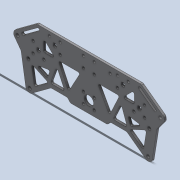
# Autodesk Inventor part: HeadTongueMount2
Saved by Autodesk Inventor 2020 (Build 240168000, 168)
## iProperties
Created: 2021-07-07
Part Number: HeadTongueMount2
Material: Generic
Document SubType Name: Sheet Metal
Designer: Val
Density: 1 g/cm^3
Sheet Metal Rule: Default
Appearance: Default
Author: Val
Autodesk Inventor part; units mm, degrees
ref_plane "YZ Plane" through (0, 0, 0) normal (1, 0, 0) x (0, 1, 0)
ref_plane "XZ Plane" through (0, 0, 0) normal (0, 1, 0) x (-1, 0, 0)
ref_plane "XY Plane" through (0, 0, 0) normal (0, 0, 1) x (1, 0, 0)
sketch "Base" plane through (0, 0, 0) normal (0, 0, 1) x (1, 0, 0)
  line L0 (97.0477, -15.5492) -> (74.2641, 1.2707)
  arc A0 (76.6398, 4.4888) -> (74.2641, 1.2707) centre (75.4519, 2.8798) ccw
  line L1 (76.6398, 4.4888) -> (99.4234, -12.3312)
  arc A1 (97.0477, -15.5492) -> (99.4234, -12.3312) centre (98.2355, -13.9402) ccw
  line L2 (-74.2641, 1.2707) -> (-97.0477, -15.5492)
  arc A2 (-99.4234, -12.3312) -> (-97.0477, -15.5492) centre (-98.2355, -13.9402) ccw
  line L3 (-99.4234, -12.3312) -> (-76.6398, 4.4888)
  arc A3 (-74.2641, 1.2707) -> (-76.6398, 4.4888) centre (-75.4519, 2.8798) ccw
  line L4 (67.5519, -9.1185) -> (67.5519, -20.0701)
  arc A4 (65.5519, -22.0701) -> (67.5519, -20.0701) centre (65.5519, -20.0701) ccw
  line L5 (65.5519, -22.0701) -> (54.6004, -22.0701)
  arc A5 (53.1861, -18.6559) -> (54.6004, -22.0701) centre (54.6004, -20.0701) ccw
  line L6 (53.1861, -18.6559) -> (64.1377, -7.7043)
  arc A6 (67.5519, -9.1185) -> (64.1377, -7.7043) centre (65.5519, -9.1185) ccw
  line L7 (-67.5519, -20.0701) -> (-67.5519, -9.1185)
  arc A7 (-64.1377, -7.7043) -> (-67.5519, -9.1185) centre (-65.5519, -9.1185) ccw
  line L8 (-64.1377, -7.7043) -> (-53.1861, -18.6559)
  arc A8 (-54.6004, -22.0701) -> (-53.1861, -18.6559) centre (-54.6004, -20.0701) ccw
  line L9 (-54.6004, -22.0701) -> (-65.5519, -22.0701)
  arc A9 (-67.5519, -20.0701) -> (-65.5519, -22.0701) centre (-65.5519, -20.0701) ccw
  arc A10 (51.746, -36.138) -> (48.4208, -33.6832) centre (50.0834, -34.9106) ccw
  line L10 (51.746, -36.138) -> (39.6773, -52.4858)
  arc A11 (36.3521, -50.0309) -> (39.6773, -52.4858) centre (38.0147, -51.2583) ccw
  line L11 (36.3521, -50.0309) -> (48.4208, -33.6832)
  arc A12 (26.5915, -49.1395) -> (29.9167, -51.5944) centre (28.2541, -50.3669) ccw
  line L12 (26.5915, -49.1395) -> (41.6774, -28.7049)
  arc A13 (45.0026, -31.1597) -> (41.6774, -28.7049) centre (43.34, -29.9323) ccw
  line L13 (45.0026, -31.1597) -> (29.9167, -51.5944)
  line L14 (74.2192, -47.1822) -> (63.9766, -52.1292)
  arc A14 (61.2238, -51.0023) -> (63.9766, -52.1292) centre (63.1067, -50.3283) ccw
  line L15 (61.2238, -51.0023) -> (58.7121, -43.9862)
  arc A15 (60.9154, -41.338) -> (58.7121, -43.9862) centre (60.5951, -43.3122) ccw
  line L16 (60.9154, -41.338) -> (73.6697, -43.4071)
  arc A16 (74.2192, -47.1822) -> (73.6697, -43.4071) centre (73.3494, -45.3813) ccw
  line L17 (19.8481, -44.1612) -> (34.934, -23.7265)
  arc A17 (38.2592, -26.1813) -> (34.934, -23.7265) centre (36.5966, -24.9539) ccw
  line L18 (38.2592, -26.1813) -> (23.1733, -46.616)
  arc A18 (19.8481, -44.1612) -> (23.1733, -46.616) centre (21.5107, -45.3886) ccw
  line L19 (62.8288, -56.8412) -> (82.3938, -47.7351)
  arc A19 (85.212, -49.868) -> (82.3938, -47.7351) centre (83.2377, -49.5483) ccw
  line L20 (85.212, -49.868) -> (81.8058, -70.9034)
  arc A20 (78.6436, -72.1927) -> (81.8058, -70.9034) centre (79.8315, -70.5837) ccw
  line L21 (78.6436, -72.1927) -> (62.4849, -60.2635)
  arc A21 (62.8288, -56.8412) -> (62.4849, -60.2635) centre (63.6727, -58.6545) ccw
  arc A22 (-48.4208, -33.6832) -> (-51.746, -36.138) centre (-50.0834, -34.9106) ccw
  line L22 (-48.4208, -33.6832) -> (-36.3521, -50.0309)
  arc A23 (-39.6773, -52.4858) -> (-36.3521, -50.0309) centre (-38.0147, -51.2583) ccw
  line L23 (-39.6773, -52.4858) -> (-51.746, -36.138)
  arc A24 (-29.9167, -51.5944) -> (-26.5915, -49.1395) centre (-28.2541, -50.3669) ccw
  line L24 (-29.9167, -51.5944) -> (-45.0026, -31.1597)
  arc A25 (-41.6774, -28.7049) -> (-45.0026, -31.1597) centre (-43.34, -29.9323) ccw
  line L25 (-41.6774, -28.7049) -> (-26.5915, -49.1395)
  line L26 (-63.9766, -52.1292) -> (-74.2192, -47.1822)
  arc A26 (-73.6697, -43.4071) -> (-74.2192, -47.1822) centre (-73.3494, -45.3813) ccw
  line L27 (-73.6697, -43.4071) -> (-60.9154, -41.338)
  arc A27 (-58.7121, -43.9862) -> (-60.9154, -41.338) centre (-60.5951, -43.3122) ccw
  line L28 (-58.7121, -43.9862) -> (-61.2238, -51.0023)
  arc A28 (-63.9766, -52.1292) -> (-61.2238, -51.0023) centre (-63.1067, -50.3283) ccw
  line L29 (-34.934, -23.7265) -> (-19.8481, -44.1612)
  arc A29 (-23.1733, -46.616) -> (-19.8481, -44.1612) centre (-21.5107, -45.3886) ccw
  line L30 (-23.1733, -46.616) -> (-38.2592, -26.1813)
  arc A30 (-34.934, -23.7265) -> (-38.2592, -26.1813) centre (-36.5966, -24.9539) ccw
  line L31 (-82.3938, -47.7351) -> (-62.8288, -56.8412)
  arc A31 (-62.4849, -60.2635) -> (-62.8288, -56.8412) centre (-63.6727, -58.6545) ccw
  line L32 (-62.4849, -60.2635) -> (-78.6436, -72.1927)
  arc A32 (-81.8058, -70.9034) -> (-78.6436, -72.1927) centre (-79.8315, -70.5837) ccw
  line L33 (-81.8058, -70.9034) -> (-85.212, -49.868)
  arc A33 (-82.3938, -47.7351) -> (-85.212, -49.868) centre (-83.2377, -49.5483) ccw
  line L34 (111.4533, -16.2403) -> (112.2956, -21.8341)
  line L35 (77.5089, 8.8191) -> (111.4533, -16.2403)
  line L36 (39.5858, 8.8191) -> (77.5089, 8.8191)
  line L37 (10, -32.979) -> (39.5858, 8.8191)
  line L38 (-10, -32.979) -> (10, -32.979)
  line L39 (-39.5858, 8.8191) -> (-10, -32.979)
  line L40 (-77.5089, 8.8191) -> (-39.5858, 8.8191)
  line L41 (-111.4533, -16.2403) -> (-77.5089, 8.8191)
  line L42 (-112.2956, -21.8341) -> (-111.4533, -16.2403)
  line L43 (-101.0503, -37.0666) -> (-112.2956, -21.8341)
  line L44 (-93.5698, -83.2627) -> (-101.0503, -37.0666)
  line L45 (-87.3317, -85.8062) -> (-93.5698, -83.2627)
  line L46 (-56.3345, -62.9226) -> (-87.3317, -85.8062)
  line L47 (-31.5391, -62.9226) -> (-56.3345, -62.9226)
  line L48 (-28, -67.9226) -> (-31.5391, -62.9226)
  line L49 (28, -67.9226) -> (-28, -67.9226)
  line L50 (31.5391, -62.9226) -> (28, -67.9226)
  line L51 (56.3345, -62.9226) -> (31.5391, -62.9226)
  line L52 (87.3317, -85.8062) -> (56.3345, -62.9226)
  line L53 (93.5698, -83.2627) -> (87.3317, -85.8062)
  line L54 (101.0503, -37.0666) -> (93.5698, -83.2627)
  line L55 (112.2956, -21.8341) -> (101.0503, -37.0666)
  arc A34 (73.6369, -26.0822) -> (73.6369, -20.7232) centre (74.9862, -23.4027) ccw
  arc A35 (72.5062, -25.0907) -> (73.6369, -26.0822) centre (73.5062, -25.0907) ccw
  line L56 (72.5062, -21.7146) -> (72.5062, -25.0907)
  arc A36 (73.6369, -20.7232) -> (72.5062, -21.7146) centre (73.5062, -21.7146) ccw
  circle A37 centre (82.9862, -15.4027) radius 2
  circle A38 centre (82.9862, -31.4027) radius 2
  circle A39 centre (66.9862, -31.4027) radius 2
  circle A40 centre (-42.6898, -13.1809) radius 2
  arc A41 (-52.039, -7.8604) -> (-52.039, -2.5014) centre (-50.6898, -5.1809) ccw
  arc A42 (-53.1698, -6.869) -> (-52.039, -7.8604) centre (-52.1698, -6.869) ccw
  line L57 (-53.1698, -3.4928) -> (-53.1698, -6.869)
  arc A43 (-52.039, -2.5014) -> (-53.1698, -3.4928) centre (-52.1698, -3.4928) ccw
  circle A44 centre (-42.6898, 2.8191) radius 2
  circle A45 centre (-58.6898, 2.8191) radius 2
  circle A46 centre (-82.9859, -31.4027) radius 2
  arc A47 (-76.3351, -20.7232) -> (-77.4659, -21.7146) centre (-76.4659, -21.7146) ccw
  arc A48 (-76.3351, -26.0822) -> (-76.3351, -20.7232) centre (-74.9859, -23.4027) ccw
  arc A49 (-77.4659, -25.0907) -> (-76.3351, -26.0822) centre (-76.4659, -25.0907) ccw
  line L58 (-77.4659, -21.7146) -> (-77.4659, -25.0907)
  circle A50 centre (-66.9859, -31.4027) radius 2
  circle A51 centre (-82.9859, -15.4027) radius 2
  circle A52 centre (42.6901, -13.1809) radius 2
  arc A53 (48.2101, -6.869) -> (49.3409, -7.8604) centre (49.2101, -6.869) ccw
  line L59 (48.2101, -3.4928) -> (48.2101, -6.869)
  arc A54 (49.3409, -2.5014) -> (48.2101, -3.4928) centre (49.2101, -3.4928) ccw
  arc A55 (49.3409, -7.8604) -> (49.3409, -2.5014) centre (50.6901, -5.1809) ccw
  circle A56 centre (42.6901, 2.8191) radius 2
  circle A57 centre (58.6901, 2.8191) radius 2
  circle A58 centre (-88.1853, -78.9786) radius 2.5
  circle A59 centre (-106.2807, -19.8795) radius 2.5
  circle A60 centre (88.1853, -78.9786) radius 2.5
  circle A61 centre (106.2807, -19.8795) radius 2.5
  circle A62 centre (90.0071, -41.923) radius 2.5
  circle A63 centre (-90.0071, -41.923) radius 2.5
  line L60 (-157.2139, 0) -> (157.2139, 0)
  line L61 (0, -104.7313) -> (0, 27.7442)
  point P0 (0, 0)
  point P1 (0, 0)
  dimension "d0" = 5
  dimension "d1" = 2
  dimension "d2" = 3
  dimension "d3" = 1
  dimension "d4" = 2.0666
  dimension "d5" = 109.697
  dimension "d6" = 36.437
  dimension "d7" = 25.78
  dimension "d8" = 9.215
  dimension "d9" = 80.802
  dimension "d10" = 24.959
  dimension "d11" = 36.437
  dimension "d12" = 8.563
  dimension "d13" = 9.198
  dimension "d14" = 67.817
  dimension "d15" = 64.221
  dimension "d16" = 90
  dimension "d17" = 65.041
  dimension "d18" = 19.697
  dimension "d19" = 80.785
  dimension "d20" = 90
  dimension "d21" = 45
  dimension "d22" = 90
  dimension "d23" = 35.292
  dimension "d24" = 35.292
  dimension "d25" = 67.817
  dimension "d26" = 8.563
  dimension "d27" = 72.5062
  dimension "d28" = 67.5519
  dimension "d29" = 48.2101
  dimension "d30" = 67.9226
  dimension "d31" = 53.1698
  dimension "d32" = 67.5519
  dimension "d33" = 77.4659
  dimension "d34" = 32.979
  dimension "d35" = 62.9226
  dimension "d36" = 22.0701
  dimension "d37" = 8.8191
  dimension "d38" = 40.2175
  dimension "d39" = 48.5995
  dimension "d40" = 56.9815
  dimension "d41" = 13.5884
  dimension "d42" = 62.2934
  dimension "d43" = 56.5013
  dimension "d44" = 8
  dimension "d45" = 34.8804
  dimension "d46" = 8.382
  dimension "d47" = 16.764
  dimension "d48" = 56.9815
  dimension "d49" = 34.8804
  dimension "d50" = 5.7922
  dimension "d51" = 62.2934
  dimension "d52" = 70.2935
  dimension "d53" = 13.5884
  dimension "d54" = 23.1694
  dimension "d55" = 47.6687
  dimension "d56" = 49.5165
  dimension "d57" = 48.2443
  dimension "d58" = 53.0704
  dimension "d59" = 6.3912
  dimension "d60" = 22.0701
  dimension "d61" = 11.7056
  dimension "d62" = 107.5636
  dimension "d63" = 56.2253
  measures "d0" diameter of A61
  measures "d1" radius of A1
  measures "d2" radius of A34
  measures "d3" radius of A36
  measures "d4" radius of A10
  measures "d5" angle of L60 L28
  measures "d6" angle of L60 L32
  measures "d7" angle of L60 L26
  measures "d8" angle of L60 L27
  measures "d9" angle of L60 L33
  measures "d10" angle of L60 L31
  measures "d11" angle of L55 L61
  measures "d12" angle of L34 L61
  measures "d13" angle of L54 L61
  measures "d14" angle of L53 L61
  measures "d15" angle of L14 L61
  measures "d16" angle of L5 L61
  measures "d17" angle of L19 L61
  measures "d18" angle of L15 L61
  measures "d19" angle of L16 L61
  measures "d20" angle of L51 L61
  measures "d21" angle of L6 L61
  measures "d22" angle of L36 L61
  measures "d23" angle of L50 L61
  measures "d24" angle of L48 L61
  measures "d25" angle of L45 L61
  measures "d26" angle of L42 L61
  measures "d27" distance between parallel lines of L56 L61
  measures "d28" distance between parallel lines of L4 L61
  measures "d29" distance between parallel lines of L59 L61
  measures "d30" distance between parallel lines of L49 L60
  measures "d31" distance between parallel lines of L57 L61
  measures "d32" distance between parallel lines of L7 L61
  measures "d33" distance between parallel lines of L58 L61
  measures "d34" distance between parallel lines of L38 L60
  measures "d35" distance between parallel lines of L47 L60
  measures "d36" distance between parallel lines of L9 L60
  measures "d37" distance between parallel lines of L40 L60
  measures "d38" distance between parallel lines of L10 L55
  measures "d39" distance between parallel lines of L13 L55
  measures "d40" distance between parallel lines of L18 L55
  measures "d41" distance between parallel lines of L54 L20
  measures "d42" distance between parallel lines of L0 L52
  measures "d43" distance between parallel lines of L0 L21
  measures "d44" distance between parallel lines of L0 L35
  measures "d45" distance between parallel lines of L50 L37
  measures "d46" distance between parallel lines of L24 L30
  measures "d47" distance between parallel lines of L30 L23
  measures "d48" distance between parallel lines of L30 L43
  measures "d49" distance between parallel lines of L48 L39
  measures "d50" distance between parallel lines of L46 L32
  measures "d51" distance between parallel lines of L2 L46
  measures "d52" distance between parallel lines of L46 L41
  measures "d53" distance between parallel lines of L44 L33
  measures "d54" distance from line of L60.end L55
  measures "d55" distance from line of L60.end L34
  measures "d56" distance from line of L60.end L54
  measures "d57" distance from line of L60.end L0
  measures "d58" distance from line of L60.end L53
  measures "d59" distance from line of L60.end L14
  measures "d60" distance from line of L60.end L5
  measures "d61" distance from line of L60.end L19
  measures "d62" distance from line of L60.end L15
  measures "d63" distance from line of L60.end L16
extrude "Plate1" add sketch "Base" along normal blind 3.175 contours A1 L1 L60 L35 L34 L55 L54 L53 L52 L51 L50 L49 L61 L38 L37 L0 | L60 L37 L36 L35 L1 A0 L0 | L61 L49 L48 L47 L46 L45 L44 L43 L42 L41 L60 L3 A2 L2 L39 L38 | L60 L2 A3 L3 L41 L40 L39 | L10 A11 L11 A10 | L12 A13 L13 A12 | L17 A17 L18 A18 | L22 A23 L23 A22 | L24 A25 L25 A24 | L29 A29 L30 A30
fillet "BaseFilletsFeature" radius 4 22 edges at (-77.5089, 8.8191, 1.5875) (-39.5858, 8.8191, 1.5875) (-10, -32.979, 1.5875) (-111.4533, -16.2403, 1.5875) (-112.2956, -21.8341, 1.5875) (-101.0503, -37.0666, 1.5875) (-93.5698, -83.2627, 1.5875) (-87.3317, -85.8062, 1.5875) (-56.3345, -62.9226, 1.5875) (-31.5391, -62.9226, 1.5875) (-28, -67.9226, 1.5875) (28, -67.9226, 1.5875) (31.5391, -62.9226, 1.5875) (56.3345, -62.9226, 1.5875) (87.3317, -85.8062, 1.5875) (93.5698, -83.2627, 1.5875) (101.0503, -37.0666, 1.5875) (112.2956, -21.8341, 1.5875) (111.4533, -16.2403, 1.5875) (77.5089, 8.8191, 1.5875) (39.5858, 8.8191, 1.5875) (10, -32.979, 1.5875)
sketch "NeckMount" plane through (0, 0, 0) normal (0, 0, -1) x (-1, 0, 0)
  line L0 (-41.6551, 8.8191) -> (-76.1924, 8.8191)
  line L1 (76.1924, 8.8191) -> (41.6551, 8.8191)
  line L2 (-41.6551, 8.8191) -> (41.6551, 8.8191)
  line L3 (41.6551, 8.8191) -> (12.0693, -32.979)
  line L4 (12.0693, -32.979) -> (-12.0693, -32.979)
  line L5 (-12.0693, -32.979) -> (-41.6551, 8.8191)
  line L6 (7.9307, -32.979) -> (-7.9307, -32.979)
  line L7 (38.3903, 7.1301) -> (11.1955, -31.2899)
  line L8 (-11.1955, -31.2899) -> (-38.3903, 7.1301)
  point P0 (0, 0)
sheet face with bend "NeckMountFeature" sketch "NeckMount" thickness 3.175 toward (0, 0, 1) bend radius 3.175 relief straight relief width 3.175 relief depth 1.5875
bend "Bend2"
sketch "NeckMountHoles" plane through (0, 0, 0) normal (0, 0, -1) x (-1, 0, 0)
  circle A0 centre (-7.9999, 2.8191) radius 2 projected
  circle A1 centre (8.0001, 2.8191) radius 2 projected
  circle A2 centre (-7.9999, -13.1809) radius 2 projected
  circle A3 centre (8.0001, -13.1809) radius 2 projected
  point P0 (0, 0)
hole "NeckMountHolesFeature" at (7.9999, 2.8191, 0) at (7.9999, -13.1809, 0) at (-8.0001, -13.1809, 0) at (-8.0001, 2.8191, 0) direction (0, 0, 1) diameter 4 depth 3.175 tip angle 118
sketch "Sketch7" plane through (0, 0, 0) normal (0, 0, -1) x (-1, 0, 0)
  arc A0 (6.5355, -44.6034) -> (6.0022, -43.1499) centre (8.0001, -43.2415) ccw projected
  arc A1 (6.6382, -57.7768) -> (8.0917, -57.2436) centre (8.0001, -59.2415) ccw projected
  arc A2 (-6.5352, -57.8796) -> (-6.002, -59.333) centre (-7.9999, -59.2415) ccw projected
  arc A3 (-6.638, -44.7062) -> (-8.0914, -45.2394) centre (-7.9999, -43.2415) ccw projected
  point P0 (0, 0)
hole "Hole2" at (7.9999, -43.2415, 0) at (7.9999, -59.2415, 0) at (-8.0001, -59.2415, 0) at (-8.0001, -43.2415, 0) direction (0, 0, 1) diameter 4 end through all
sketch "Sketch8" plane through (0, 0, 0) normal (0, 0, -1) x (-1, 0, 0)
  circle A0 centre (0.0001, -51.1404) radius 7
  point P0 (0, 0)
  dimension "d213" = 14
  constraints: 1 centre point, 1 other
  measures "d213" diameter of A0
extrude "Cut3" cut sketch "Sketch8" against normal blind 3.175
sketch "Sketch9" plane through (0, 0, 0) normal (0, 0, -1) x (-1, 0, 0)
  line L0 (-57.2654, -57.1304) -> (-35.7621, -57.1304)
  line L1 (-57.2654, -57.1304) -> (-47.9266, -31.0434)
  line L2 (-47.9266, -31.0434) -> (-35.7621, -57.1304)
  line L3 (-45.72, -22.0701) -> (-12.7, -22.0701)
  line L4 (-12.7, -22.0701) -> (-30.5126, -54.6826)
  line L5 (-30.5126, -54.6826) -> (-45.72, -22.0701)
  line L6 (-58.7121, -43.9862) -> (-61.2238, -51.0023) projected
  line L7 (-55.018, -62.9226) -> (-33.6085, -62.9226) projected
  line L8 (76.1924, 8.8191) -> (-76.1924, 8.8191) projected
  line L9 (-85.5251, -84.4725) -> (-57.3937, -63.7046) projected
  line L10 (-62.4849, -60.2635) -> (-78.6436, -72.1927) projected
  line L11 (-54.6004, -22.0701) -> (-65.5519, -22.0701) projected
  line L12 (-25.9307, -67.9226) -> (25.9307, -67.9226) projected
  line L13 (76.1924, 8.8191) -> (-76.1924, 8.8191) projected
  line L14 (0, 8.8191) -> (0, -67.9226) construction
  line L15 (-25.9307, -67.9226) -> (25.9307, -67.9226) projected
  line L16 (57.2654, -57.1304) -> (35.7621, -57.1304)
  line L17 (57.2654, -57.1304) -> (47.9266, -31.0434)
  line L18 (47.9266, -31.0434) -> (35.7621, -57.1304)
  line L19 (45.72, -22.0701) -> (12.7, -22.0701)
  line L20 (12.7, -22.0701) -> (30.5126, -54.6826)
  line L21 (30.5126, -54.6826) -> (45.72, -22.0701)
  line L22 (-35.7621, -57.1304) -> (-30.5126, -54.6826) construction
  point P0 (0, 0)
  dimension "d202" = 5.7922
  dimension "d203" = 5.7922
  dimension "d204" = 5.7922
  dimension "d205" = 5.7922
  dimension "d206" = 115
  dimension "d207" = 33.02
  dimension "d208" = 12.7
  constraints: 28 end point, 6 symmetric about line, 4 parallel, 2 midpoint, 1 collinear, 1 horizontal, 1 perpendicular
  measures "d202" distance between parallel lines of L9 L10
  measures "d203" distance between parallel lines of L7 L0
  measures "d204" distance between parallel lines of L5 L2
  measures "d205" distance between parallel lines of L6 L1
  measures "d206" angle of L12 L2
  measures "d207" distance of L3.start L3.end
  measures "d208" distance from line of L14 L3.end
extrude "Cut4" cut sketch "Sketch9" against normal blind 3.175
fillet "Fillet2" radius 2 12 edges at (47.9266, -31.0434, 1.5875) (57.2654, -57.1304, 1.5875) (35.7621, -57.1304, 1.5875) (45.72, -22.0701, 1.5875) (30.5126, -54.6826, 1.5875) (12.7, -22.0701, 1.5875) (-45.72, -22.0701, 1.5875) (-12.7, -22.0701, 1.5875) (-30.5126, -54.6826, 1.5875) (-57.2654, -57.1304, 1.5875) (-35.7621, -57.1304, 1.5875) (-47.9266, -31.0434, 1.5875)
sketch "Sketch10" plane through (0, 0, 0) normal (0, 0, -1) x (-1, 0, 0)
  ellipse E0 centre (-31.7499, -0.1394) end of major axis (-33.7499, -0.1394) minor radius 2 projected
  ellipse E1 centre (31.7501, -0.1394) end of major axis (29.7501, -0.1394) minor radius 2 projected
  point P0 (-31.7499, -0.1394)
  constraints: 2 other
hole "Hole3" at (31.7499, -0.1394, 0) at (-31.7501, -0.1394, 0) direction (0, 0, 1) diameter 4 end through all
equation "\"d185\" = Thickness"
equation "\"d157\" = Thickness"
equation "\"d175\" = BendRadius"
equation "\"d176\" = BendReliefWidth"
equation "\"d178\" = MinimumRemnant"
equation "\"d177\" = BendReliefDepth"
equation "\"d179\" = TransitionRadius"
equation "\"BendRadius\" = Thickness"
equation "\"BendReliefWidth\" = Thickness"
equation "\"BendReliefDepth\" = 0.5 * Thickness"
equation "\"CornerReliefSize\" = 4 * Thickness"
equation "\"MinimumRemnant\" = 2 * Thickness"
equation "\"TransitionRadius\" = BendRadius"
equation "\"JacobiRadiusSize\" = BendRadius"
equation "\"GapSize\" = Thickness"
equation "\"Thickness\" = 3.175"
body "Solid1"
